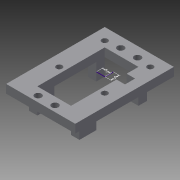
# Autodesk Inventor part: servorPlace
Saved by Autodesk Inventor 2015 (Build 190159000, 159)
## iProperties
Created: 2016-10-16
Part Number: servorPlace
Material: Generic
Document SubType Name: Modeling
Designer: Bardo91
Density: 1 g/cm^3
Appearance: Default
Author: Bardo91
Autodesk Inventor part; units mm, degrees
ref_plane "YZ Plane" through (0, 0, 0) normal (1, 0, 0) x (0, 1, 0)
ref_plane "XZ Plane" through (0, 0, 0) normal (0, 1, 0) x (-1, 0, 0)
ref_plane "XY Plane" through (0, 0, 0) normal (0, 0, 1) x (1, 0, 0)
sketch "Sketch1" plane through (0, 0, 0) normal (0, 0, 1) x (1, 0, 0)
  line L0 (0, 0) -> (-17.5, 0)
  line L1 (-17.5, 0) -> (-17.5, 17.5)
  line L2 (-17.5, 17.5) -> (17.5, 17.5)
  line L3 (-17.5, 17.5) -> (-17.5, 13.5)
  line L4 (-17.5, 13.5) -> (-13.5, 13.5)
  circle A0 centre (-13.5, 13.5) radius 1.75
  circle A1 centre (-13.5, -13.5) radius 1.75
  circle A2 centre (13.5, -13.5) radius 1.75
  circle A3 centre (13.5, 13.5) radius 1.75
  line L5 (0, 0) -> (-10, 0)
  line L6 (-10, 0) -> (-10, 10)
  line L7 (-10, 10) -> (10, 10)
  line L8 (10, 10) -> (10, -30)
  line L9 (10, -30) -> (-10, -30)
  line L10 (-10, -30) -> (-10, 0)
  line L11 (-17.5, 0) -> (-17.5, -35)
  line L12 (-17.5, -35) -> (17.5, -35)
  line L13 (17.5, -35) -> (17.5, 17.5)
  line L14 (10, 10) -> (10, 3)
  line L15 (10, 3) -> (15, 3)
  line L16 (15, 3) -> (15, -3)
  line L17 (15, -3) -> (10, -3)
  line L18 (-17.5, 17.5) -> (-17.5, 20.5)
  line L19 (-17.5, 20.5) -> (20.5, 20.5)
  line L20 (20.5, 20.5) -> (20.5, -38)
  line L21 (20.5, -38) -> (-20.5, -38)
  line L22 (-20.5, -38) -> (-20.5, 20.5)
  line L23 (-20.5, 20.5) -> (-17.5, 20.5)
  dimension "d0" = 17.5
  dimension "d1" = 17.5
  dimension "d2" = 35
  dimension "d3" = 4
  dimension "d4" = 4
  dimension "d5" = 3.5
  dimension "d8" = 360
  dimension "d10" = 10
  dimension "d11" = 10
  dimension "d12" = 20
  dimension "d13" = 40
  dimension "d14" = 20
  dimension "d15" = 35
  dimension "d16" = 7
  dimension "d17" = 5
  dimension "d18" = 6
  dimension "d19" = 3
  dimension "d20" = 38
  dimension "d21" = 58.5
  dimension "d22" = 41
  constraints: 48 end point, 15 perpendicular, 6 point on line, 4 centre point, 2 horizontal, 2 vertical, 1 coincident, 9 other
  measures "d0" distance of L0.start L0.end
  measures "d1" distance of L0.end L1.end
  measures "d2" distance of L1.end L2.end
  measures "d3" distance of L1.end L3.end
  measures "d4" distance of L3.end L4.end
  measures "d5" diameter of A0
  measures "d10" distance of L0.start L5.end
  measures "d11" distance of L5.end L6.end
  measures "d12" distance of L6.end L7.end
  measures "d13" distance of L7.end L8.end
  measures "d14" distance of L8.end L9.end
  measures "d15" distance of L0.end L11.end
  measures "d16" distance of L7.end L14.end
  measures "d17" distance of L14.end L15.end
  measures "d18" distance of L15.end L16.end
  measures "d19" distance of L1.end L18.end
  measures "d20" distance of L18.end L19.end
  measures "d21" distance of L19.end L20.end
  measures "d22" distance of L20.end L21.end
extrude "Extrusion1" add sketch "Sketch1" along normal blind 5 contours L1 L2 L13 L12 L11 | L19 L20 L21 L22 L23
sketch "Sketch2" plane through (0, 0, 0) normal (0, 0, -1) x (-1, 0, 0)
  circle A0 centre (-13.5, 13.5) radius 1.75 projected
  line L0 (-13.5, 13.5) -> (-10.5, 13.5)
  line L1 (-10.5, 13.5) -> (-12, 16.0981)
  line L2 (-12, 16.0981) -> (-13.5, 13.5)
  point P0 (0, 0)
  dimension "d25" = 3
  dimension "d26" = 3
  dimension "d27" = 60
  constraints: 6 end point, 1 horizontal
  measures "d25" distance of L0.start L0.end
  measures "d26" distance of L0.end L1.end
  measures "d27" angle of L1 L0
extrude "Extrusion2" cut sketch "Sketch2" against normal blind 2.5 contours L0 L2 A0 | A0 L2 L1 L0 picked at (-12.4952, 14.0801)
pattern_circular "Circular Pattern1" count 6 over 360 about axis through (13.5, 13.5, 0) along (0, 0, 1) of "Extrusion2"
sketch "Sketch3" plane through (0, 0, 0) normal (0, 0, -1) x (-1, 0, 0)
  line L0 (0, 0) -> (5, 0)
  line L1 (0, 0) -> (0, 5)
  dimension "d33" = 5
  dimension "d34" = 5
  constraints: 4 end point, 1 horizontal, 1 vertical
  measures "d33" distance of L0.start L0.end
  measures "d34" distance of L0.start L1.end
pattern_linear "Rectangular Pattern1" count 2 spacing 27 along (-1, 0, 0) count 2 spacing 27 along (0, -1, 0) of "Extrusion2", "Circular Pattern1"
sketch "Sketch4" plane through (0, 0, 5) normal (0, 0, 1) x (1, 0, 0)
  line L0 (-10, 10) -> (10, 10) projected
  line L1 (0, 10) -> (0, 14.5)
  line L2 (0, 14.5) -> (3, 14.5)
  line L3 (3, 14.5) -> (-3, 14.5)
  line L4 (3, 14.5) -> (5, 14.5)
  line L5 (-3, 14.5) -> (-5, 14.5)
  circle A0 centre (-5, 14.5) radius 2
  circle A1 centre (5, 14.5) radius 2
  line L6 (10, 10) -> (10, -30)
  line L7 (-10, -30) -> (10, -30) projected
  line L8 (10, 10) -> (10, -10)
  line L9 (10, -30) -> (10, -3) projected
  line L10 (10, -10) -> (0.7941, -10)
  circle A2 centre (-5, -34.5) radius 2
  circle A3 centre (5, -34.5) radius 2
  point P0 (0, 0)
  dimension "d41" = 4.5
  dimension "d42" = 3
  dimension "d43" = 6
  dimension "d44" = 2
  dimension "d45" = 2
  dimension "d46" = 4
  dimension "d47" = 4
  dimension "d48" = 20
  constraints: 16 end point, 4 centre point, 3 horizontal, 2 coincident, 2 perpendicular, 2 point on line, 2 symmetric about line, 1 midpoint, 1 vertical, 2 other
  measures "d41" distance of L1.start L1.end
  measures "d42" distance of L1.end L2.end
  measures "d43" distance of L2.end L3.end
  measures "d44" distance of L2.end L4.end
  measures "d45" distance of L3.end L5.end
  measures "d46" diameter of A0
  measures "d47" diameter of A1
  measures "d48" distance of L0.end L8.end
extrude "Extrusion3" cut sketch "Sketch4" against normal through all
sketch "Sketch5" plane through (0, 0, 0) normal (0, 0, -1) x (-1, 0, 0)
  line L0 (10, -30) -> (15, -30)
  line L1 (15, -30) -> (15, -20)
  line L2 (15, -20) -> (10, -20)
  line L3 (10, 10) -> (10, -30) projected
  line L4 (-10, -30) -> (-15, -30)
  line L5 (-15, -30) -> (-15, -20)
  line L6 (-15, -20) -> (-10, -20)
  line L7 (-10, -30) -> (-10, -3) projected
  line L8 (-10, -30) -> (-10, -20)
  line L9 (10, -20) -> (10, -30)
  line L10 (-10, 10) -> (-15, 10)
  line L11 (-15, 10) -> (-15, 5)
  line L12 (-15, 5) -> (-10, 5)
  line L13 (-10, 3) -> (-10, 10) projected
  line L14 (-10, 10) -> (-10, 5)
  line L15 (10, 10) -> (15, 10)
  line L16 (15, 10) -> (15, 5)
  line L17 (15, 5) -> (10, 5)
  line L18 (10, 10) -> (10, 5)
  point P0 (0, 0)
  dimension "d51" = 5
  dimension "d52" = 10
  dimension "d53" = 5
  dimension "d54" = 10
  dimension "d55" = 5
  dimension "d56" = 5
  dimension "d57" = 5
  dimension "d58" = 5
  constraints: 32 end point, 9 point on line, 8 perpendicular, 1 collinear, 1 horizontal, 1 parallel
  measures "d51" distance of L0.start L0.end
  measures "d52" distance of L0.end L1.end
  measures "d53" distance of L4.start L4.end
  measures "d54" distance of L4.end L5.end
  measures "d55" distance of L10.start L10.end
  measures "d56" distance of L10.end L11.end
  measures "d57" distance of L3.start L15.end
  measures "d58" distance of L15.end L16.end
extrude "Extrusion4" add sketch "Sketch5" along normal blind 10
body "Solid1"
